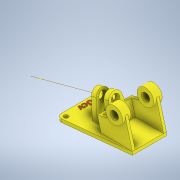
# Autodesk Inventor part: Cocei g. Janina constantina-T1
Saved by Autodesk Inventor 2022 (Build 260153000, 153)
## iProperties
Created: 2022-02-17
Part Number: Cocei g. Janina constantina-T1
Material: Steel, Carbon
Document SubType Name: Modeling
Designer: cteis
Density: 7.85363 g/cm^3
Appearance: Canary
Mass: 884 g
Surface Area: 404.883 cm^2
Volume: 112.559 cm^3
Student_ACE: Cocei g. Janina constantina
Grupa_ACE: CR-1
Tema_ACE: 1-Reper parametric
An_ACE: 2022
Author: cteis
Autodesk Inventor part; units mm, degrees
ref_plane "YZ Plane" through (0, 0, 0) normal (1, 0, 0) x (0, 1, 0)
ref_plane "XZ Plane" through (0, 0, 0) normal (0, 1, 0) x (-1, 0, 0)
ref_plane "XY Plane" through (0, 0, 0) normal (0, 0, 1) x (1, 0, 0)
sketch "Sketch4" plane through (0, 0, 0) normal (0, 0, 1) x (1, 0, 0)
  line L0 (-28.9877, 0) -> (173.9264, 0) projected
  line L1 (-29.4372, -7.8877) -> (176.6233, 47.3261) projected
  line L2 (101.2142, 39.5436) -> (109.9075, 41.8729)
  line L3 (109.9075, 41.8729) -> (118.9662, 8.0655)
  line L4 (118.9662, 8.0655) -> (132.4891, 11.689)
  line L5 (132.4891, 11.689) -> (123.4305, 45.4964)
  line L6 (123.4305, 45.4964) -> (132.1238, 47.8258)
  line L7 (132.1238, 47.8258) -> (144.9387, 0)
  line L8 (144.9387, 0) -> (111.8098, 0)
  line L9 (111.8098, 0) -> (101.2142, 39.5436)
  point P0 (0, 0)
  dimension "d31" = 9
  dimension "d32" = 35
  dimension "d34" = 12
  dimension "d35" = 117
  dimension "d36" = 9
  dimension "d37" = 14
  constraints: 16 end point, 5 perpendicular, 2 point on line, 1 collinear, 1 horizontal, 1 parallel
  measures "d31" distance of L2.start L2.end
  measures "d32" distance of L2.end L3.end
  measures "d34" distance between parallel lines of L1 L6
  measures "d35" distance from line of point (0, 0) L3
  measures "d36" distance of L5.end L6.end
  measures "d37" distance of L3.end L4.end
extrude "Extrusion1" add sketch "Sketch4" along normal mid plane 50 contours L9 L1 L3 L4 L5 L7 L0 | L9 L2 L3 L1 | L1 L5 L6 L7
sketch "Sketch5" plane through (111.8098, 0, -25) normal (-0.9659258, -0.258819, 0) x (0, 0, 1)
  line L0 (25, 64.8401) -> (25, -46.4712) projected
  line L1 (0, 40.9385) -> (50, 40.9385) projected
  line L2 (0, -8.5744) -> (50, -8.5744) projected
  line L3 (1.57, -23.5744) -> (48.43, -23.5744)
  line L4 (1.57, -23.5744) -> (13.2622, 31.4335)
  line L5 (48.43, -23.5744) -> (36.7378, 31.4335)
  arc A0 (36.7378, 31.4335) -> (13.2622, 31.4335) centre (25, 28.9385) ccw
  point P0 (25, 28.9385)
  dimension "d40" = 12
  dimension "d41" = 78
  dimension "d42" = 78
  dimension "d43" = 15
  constraints: 6 end point, 3 tangent, 2 point on circle, 1 centre point, 1 horizontal, 1 point on line
  measures "d40" radius of A0
  measures "d41" angle of L4 L3
  measures "d42" angle of L5 L3
  measures "d43" distance between parallel lines of L2 L3
extrude "Extrusion2" cut sketch "Sketch5" against normal blind 50 keep common part
sketch "Sketch6" plane through (0, 0, 0) normal (0, 0, 1) x (1, 0, 0)
  line L0 (-28.9877, 0) -> (173.9264, 0) projected
  line L1 (-29.4372, -7.8877) -> (176.6233, 47.3261) projected
  line L2 (182.56, 48.9168) -> (195.6672, 0)
  line L3 (195.6672, 0) -> (139.7623, 0)
  line L4 (139.7623, 0) -> (132.9832, 25.3)
  line L5 (132.9832, 25.3) -> (156.1654, 31.5117)
  line L6 (156.1654, 31.5117) -> (153.5822, 41.1522)
  line L7 (153.5822, 41.1522) -> (182.56, 48.9168)
  line L8 (118.9662, 8.0655) -> (132.4891, 11.689) projected
  line L9 (134.5839, 38.6446) -> (144.9387, 0) projected
  line L10 (132.1238, 47.8258) -> (134.5839, 38.6446) projected
  line L11 (132.4891, 11.689) -> (125.8905, 36.3152) projected
  point P0 (0, 0)
  point P1 (168.0711, 45.0345)
  point P2 (195.6672, 0)
  dimension "d46" = 30
  dimension "d47" = 25.3
  dimension "d48" = 49
  dimension "d52" = 5
  constraints: 12 end point, 4 perpendicular, 1 collinear, 1 horizontal, 1 midpoint, 1 parallel, 1 point on line
  measures "d46" distance of L6.end L2.start
  measures "d47" vertical distance of L3.end L4.end
  measures "d48" distance between parallel lines of L10 L2
  measures "d52" distance between parallel lines of L9 L4
extrude "Extrusion3" add sketch "Sketch6" along normal mid plane 61 contours L4 L5 L9 L0 | L9 L5 L6 L1 L7 L2 L3 L0
sketch "Sketch7" plane through (153.5822, 41.1522, 30.5) normal (-0.258819, 0.9659258, 0) x (0.9659258, 0.258819, 0)
  point P0 (-159, 30.5)
sketch "Sketch8" plane through (153.5822, 41.1522, 30.5) normal (-0.258819, 0.9659258, 0) x (0.9659258, 0.258819, 0)
  line L0 (35, 56) -> (-19, 56)
  line L1 (-19, 56) -> (-19, 5)
  line L2 (-19, 5) -> (35, 5)
  line L3 (35, 5) -> (35, 56)
  line L4 (30, 0) -> (0, 0) projected
  line L5 (0, 61) -> (30, 61) projected
  line L6 (-24, 44.8895) -> (-24, 61) projected
  line L7 (30, 61) -> (30, 0) projected
  point P0 (-159, 30.5)
  dimension "d55" = 5
  dimension "d56" = 5
  dimension "d57" = 5
  dimension "d58" = 5
  constraints: 8 end point, 2 parallel, 1 horizontal, 1 perpendicular
  measures "d55" distance between parallel lines of L2 L4
  measures "d56" distance between parallel lines of L5 L0
  measures "d57" distance between parallel lines of L6 L1
  measures "d58" distance between parallel lines of L3 L7
extrude "Extrusion4" cut sketch "Sketch8" against normal through all
sketch "Sketch9" plane through (0, 0, 0) normal (0, 0, 1) x (1, 0, 0)
  line L0 (153.5822, 41.1522) -> (182.56, 48.9168) projected
  circle A0 centre (168.0711, 45.0345) radius 15
  line L1 (182.56, 48.9168) -> (195.6672, 0) projected
  point P0 (0, 0)
  dimension "d65" = 30
  constraints: 1 centre point, 1 midpoint, 1 tangent
  measures "d65" diameter of A0
extrude "Extrusion5" add sketch "Sketch9" along normal mid plane 71
sketch "Sketch10" plane through (0, 0, 0) normal (0, 0, 1) x (1, 0, 0)
  circle A0 centre (168.0711, 45.0345) radius 19.5
  circle A1 centre (168.0711, 45.0345) radius 15 projected
  point P0 (0, 0)
  dimension "d68" = 39
  constraints: 1 centre point, 1 concentric
  measures "d68" diameter of A0
extrude "Extrusion6" cut sketch "Sketch10" along normal mid plane 41 contours A0 | A1
sketch "Sketch12" plane through (0, 0, 0) normal (0, 1, 0) x (-1, 0, 0)
  line L0 (-234.8006, 0) -> (39.1334, 0) projected
  line L1 (-72.8641, -35) -> (-72.8641, 35)
  arc A0 (-82.6672, -42.7941) -> (-72.8641, -35) centre (-80.8641, -35) ccw
  arc A1 (-72.8641, 35) -> (-81.3873, 42.9829) centre (-80.8641, 35) ccw
  line L2 (-195.6672, -30.5) -> (-195.6672, -25.5) projected
  line L3 (-195.6672, 25.5) -> (-195.6672, 30.5) projected
  line L4 (-81.3873, 42.9829) -> (-195.6672, 30.5)
  line L5 (-195.6672, 30.5) -> (-195.6672, -30.5)
  line L6 (-195.6672, -30.5) -> (-82.6672, -42.7941)
  point P0 (0, 0)
  dimension "d83" = 8
  dimension "d84" = 8
  dimension "d86" = 113
  dimension "d87" = 35
  dimension "d88" = 35
  dimension "d89" = 70
  constraints: 8 end point, 4 point on circle, 2 centre point, 2 tangent, 2 vertical
  measures "d83" radius of A0
  measures "d84" radius of A1
  measures "d86" horizontal distance of L2.start L6.end
  measures "d87" distance from line of A0.centre L0
  measures "d88" distance from line of L0 A1.centre
  measures "d89" distance of L1.start L1.end
extrude "Extrusion7" add sketch "Sketch12" against normal blind 6
sketch "Sketch13" plane through (168.0711, 45.0345, 35.5) normal (0, 0, 1) x (1, 0, 0)
  point P0 (-168.0711, -45.0345)
  point P1 (0.2725, -0.1839)
hole "Hole1" at (168.3436, 44.8506, 35.5) direction (0, 0, -1) diameter 15 end through all
sketch "Sketch14" plane through (104.32, 27.9525, 0) normal (-0.9659258, -0.258819, 0) x (0, 0, 1)
  point P0 (0, 0)
  point P1 (0, 0)
  constraints: 1 coincident
hole "Hole2" at (104.32, 27.9525, 0) direction (0.9659258, 0.258819, 0) diameter 15 end through all both
sketch "Sketch15" plane through (0, 0, 0) normal (0, 1, 0) x (1, 0, 0)
  point P0 (0, 0)
  point P1 (80.96, 34.7751)
  point P2 (81.8517, -35.6668)
hole "Hole3" at (80.96, 0, -34.7751) at (81.8517, 0, 35.6668) direction (0, -1, 0) diameter 8 end through all both
sketch "Sketch18" plane through (0, 0, 0) normal (0, 1, 0) x (1, 0, 0)
  line L0 (87.8641, 14.5) -> (87.8641, -14.5) construction
  line L1 (87.8641, -14.5) -> (76.8641, -14.5) construction
  line L2 (76.8641, -14.5) -> (76.8641, 14.5) construction
  line L3 (76.8641, 14.5) -> (87.8641, 14.5) construction
  line L4 (72.8641, 35) -> (72.8641, -35) projected
  spline S0 degree 2 poles (77.2587, 7.6053) (77.2587, 9.6232) (79.2036, 11.795) (81.0837, 11.795) knots 0 0 0 1 2 2 2
  line L5 (81.0837, 11.795) -> (87.4694, 11.795)
  line L6 (87.4694, 11.795) -> (87.4694, 9.2828)
  line L7 (87.4694, 9.2828) -> (81.2296, 9.2828)
  spline S1 degree 2 poles (81.2296, 9.2828) (80.1842, 9.2828) (79.1631, 8.4968) (79.1631, 7.6053) knots 0 0 0 1 2 2 2
  spline S2 degree 2 poles (79.1631, 7.6053) (79.1631, 6.7382) (80.1437, 5.9279) (81.2296, 5.9279) knots 0 0 0 1 2 2 2
  line L8 (81.2296, 5.9279) -> (87.4694, 5.9279)
  line L9 (87.4694, 5.9279) -> (87.4694, 3.4157)
  line L10 (87.4694, 3.4157) -> (81.0918, 3.4157)
  spline S3 degree 2 poles (81.0918, 3.4157) (79.2441, 3.4157) (77.2587, 5.5308) (77.2587, 7.6053) knots 0 0 0 1 2 2 2
  spline S4 degree 2 poles (77.2668, -2.0705) (77.2668, -1.1386) (77.7368, 0.4092) (78.2231, 0.9846) knots 0 0 0 1 2 2 2
  spline S5 degree 2 poles (78.2231, 0.9846) (78.7174, 1.5438) (80.2004, 2.1759) (81.2052, 2.1759) knots 0 0 0 1 2 2 2
  spline S6 degree 2 poles (81.2052, 2.1759) (82.2911, 2.1759) (83.8065, 1.4951) (84.2928, 0.9036) knots 0 0 0 1 2 2 2
  spline S7 degree 2 poles (84.2928, 0.9036) (84.7628, 0.3444) (85.2166, -1.1791) (85.2166, -2.0057) knots 0 0 0 1 2 2 2
  spline S8 degree 2 poles (85.2166, -2.0057) (85.2166, -2.6297) (84.9249, -3.8776) (84.6088, -4.5097) knots 0 0 0 1 2 2 2
  line L11 (84.6088, -4.5097) -> (82.5991, -4.5097)
  line L12 (82.5991, -4.5097) -> (82.5991, -4.2099)
  spline S9 degree 2 poles (82.5991, -4.2099) (82.7368, -4.064) (83.061, -3.6588) (83.1907, -3.4157) knots 0 0 0 1 2 2 2
  spline S10 degree 2 poles (83.1907, -3.4157) (83.3365, -3.1564) (83.531, -2.5162) (83.531, -2.1191) knots 0 0 0 1 2 2 2
  spline S11 degree 2 poles (83.531, -2.1191) (83.531, -1.2196) (82.2749, -0.231) (81.2052, -0.231) knots 0 0 0 1 2 2 2
  spline S12 degree 2 poles (81.2052, -0.231) (80.0707, -0.231) (78.9524, -1.2844) (78.9524, -2.1596) knots 0 0 0 1 2 2 2
  spline S13 degree 2 poles (78.9524, -2.1596) (78.9524, -2.6053) (79.155, -3.2699) (79.3009, -3.513) knots 0 0 0 1 2 2 2
  spline S14 degree 2 poles (79.3009, -3.513) (79.4386, -3.748) (79.7466, -4.0883) (79.8681, -4.2099) knots 0 0 0 1 2 2 2
  line L13 (79.8681, -4.2099) -> (79.8681, -4.5097)
  line L14 (79.8681, -4.5097) -> (77.8503, -4.5097)
  spline S15 degree 2 poles (77.8503, -4.5097) (77.7612, -4.3071) (77.5343, -3.7804) (77.4613, -3.5049) knots 0 0 0 1 2 2 2
  spline S16 degree 2 poles (77.4613, -3.5049) (77.3641, -3.1645) (77.2668, -2.5648) (77.2668, -2.0705) knots 0 0 0 1 2 2 2
  line L15 (85.014, -12.6864) -> (77.4694, -9.9797)
  line L16 (77.4694, -9.9797) -> (77.4694, -7.4109)
  line L17 (77.4694, -7.4109) -> (85.014, -4.7285)
  line L18 (85.014, -4.7285) -> (85.014, -7.2002)
  line L19 (85.014, -7.2002) -> (80.0302, -8.7399)
  line L20 (80.0302, -8.7399) -> (85.014, -10.2634)
  line L21 (85.014, -10.2634) -> (85.014, -12.6864)
  point P0 (0, 0)
  point P1 (72.8641, 0)
  point P2 (76.8641, 0)
  dimension "d118" = 11
  dimension "d119" = 15
  dimension "d120" = 29
  constraints: 2 midpoint, 1 horizontal alignment, 1 parallel, 2 other
  measures "d118" distance of L0.end L1.end
  measures "d119" distance between parallel lines of L4 L0
  measures "d120" distance of L1.end L2.end
emboss "Emboss1" sketch "Sketch18" operation add depth 1 direction (0, -1, 0)
body "Solid1"
